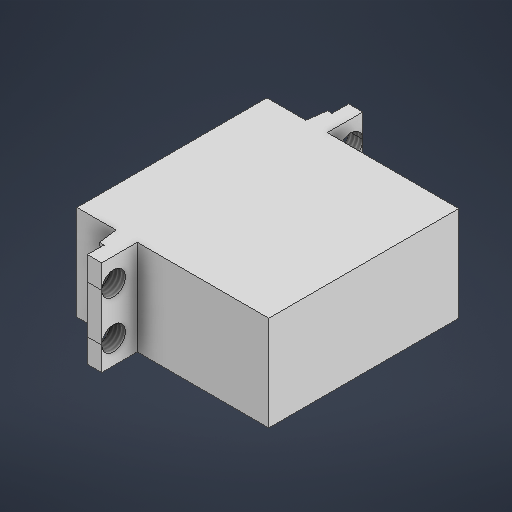
# Autodesk Inventor part: Servo
Saved by Autodesk Inventor 2026.1 (Build 301233000, 233)
## iProperties
Created: 2026-07-12
Part Number: Servo
Material: Generic
Document SubType Name: Modeling
Designer: ankit
Density: 1 g/cm^3
Appearance: Default
Author: ankit
Autodesk Inventor part; units mm, degrees
ref_plane "YZ Plane" through (0, 0, 0) normal (1, 0, 0) x (0, 1, 0)
ref_plane "XZ Plane" through (0, 0, 0) normal (0, 1, 0) x (-1, 0, 0)
ref_plane "XY Plane" through (0, 0, 0) normal (0, 0, 1) x (1, 0, 0)
sketch "Sketch1" plane through (0, 0, 0) normal (0, 1, 0) x (-1, 0, 0)
  line L0 (20.2, 20) -> (-20.2, 20)
  line L1 (-20.2, 20) -> (-20.2, -20)
  line L2 (-20.2, -20) -> (20.2, -20)
  line L3 (20.2, -20) -> (20.2, 20)
  line L4 (20.2, 20) -> (-20.2, -20) construction
  line L5 (-20.2, 20) -> (20.2, -20) construction
  line L6 (-20.2, 20) -> (7.5, 20)
  line L7 (7.5, 20) -> (7.5, 27.5)
  line L8 (7.5, 27.5) -> (10.5, 27.5)
  line L9 (10.5, 27.5) -> (10.5, 20)
  line L10 (10.5, 24) -> (11.4512, 24)
  line L11 (11.4512, 24) -> (12, 20)
  line L12 (20.2, 0) -> (-20.2, 0)
  line L13 (7.5, -20) -> (7.5, -27.5)
  line L14 (7.5, -27.5) -> (10.5, -27.5)
  line L15 (10.5, -27.5) -> (10.5, -20)
  line L16 (10.5, -24) -> (11.4512, -24)
  line L17 (11.4512, -24) -> (12, -20)
  line L18 (-20.2, -20) -> (-15.2, -20)
  line L19 (-15.2, -20) -> (-15.2, -23)
  line L20 (-15.2, -23) -> (-13.2, -23)
  line L21 (-13.2, -23) -> (-13.2, -20)
  point P0 (0, 0)
  dimension "d0" = 40.4
  dimension "d1" = 40
  dimension "d2" = 27.7
  dimension "d3" = 7.5
  dimension "d4" = 3
  dimension "d5" = 5
  dimension "d6" = 2
  constraints: 44 end point, 8 perpendicular, 7 point on line, 7 symmetric about line, 4 midpoint, 2 parallel, 1 horizontal
  measures "d0" distance of L2.end L1.end
  measures "d1" distance of L1.end L0.end
  measures "d2" distance of L0.end L6.end
  measures "d3" distance of L6.end L7.end
  measures "d4" distance of L7.end L8.end
  measures "d5" distance of L1.end L18.end
  measures "d6" distance of L19.end L20.end
extrude "Extrusion1" add sketch "Sketch1" along normal blind 20
sketch "Sketch3" plane through (-20.2, 0, -20) normal (-1, 0, 0) x (0, 0, 1)
  circle A0 centre (31, 10) radius 1.5
  line L0 (47.5, 0) -> (47.5, 20) projected
  line L1 (47.5, 10) -> (-7.5, 10)
  line L2 (-7.5, 0) -> (-7.5, 20) projected
  line L3 (20, 0) -> (20, 20)
  line L4 (0, 20) -> (40, 20) projected
  circle A1 centre (45, 5) radius 2.5
  circle A2 centre (45, 15) radius 2.5
  circle A3 centre (-5, 5) radius 2.5
  circle A4 centre (-5, 15) radius 2.5
  line L5 (45, 5) -> (45, 5)
  dimension "d24" = 0
  constraints: 6 end point, 5 centre point, 3 midpoint, 3 symmetric about line, 1 vertical, 3 other
  measures "d24" distance of L5.start L5.end
sketch "Sketch4" plane through (15.2, 0, -23) normal (0, 0, -1) x (-1, 0, 0)
  line L0 (0, 0) -> (0, 20) projected
  line L1 (4, 25) -> (0, 25)
  line L2 (0, 25) -> (0, 15)
  line L3 (0, 15) -> (4, 15)
  line L4 (4, 15) -> (4, 25)
  line L5 (2, 0) -> (2, 20) projected
  line L6 (4, 25) -> (0, 15) construction
  line L7 (0, 25) -> (4, 15) construction
  line L8 (4, -5) -> (0, -5)
  line L9 (0, -5) -> (0, 5)
  line L10 (0, 5) -> (4, 5)
  line L11 (4, 5) -> (4, -5)
  line L12 (4, -5) -> (0, 5) construction
  line L13 (0, -5) -> (4, 5) construction
  point P0 (15.2, 0)
  constraints: 24 end point, 4 midpoint, 4 parallel, 2 horizontal, 2 perpendicular, 2 point on line
extrude "Extrusion4" cut sketch "Sketch4" against normal blind 3 contours L0 L10 L11 L8 L9 | L0 L2 L1 L4 L3
extrude "Extrusion5" cut sketch "Sketch3" against normal blind 15 contours A3 | A4 | A2 | A1
extrude "Extrusion6" add sketch "Sketch3" along normal blind 5 contours L1 A0 | A0 L1
thread "Thread1" size "M5x0.8" class "6H" standard "ANSI Metric M Profile" full length
thread "Thread2" size "M5x0.8" class "6H" standard "ANSI Metric M Profile" full length
thread "Thread3" size "M5x0.8" class "6H" standard "ANSI Metric M Profile" full length
thread "Thread4" size "M5x0.8" class "6H" standard "ANSI Metric M Profile" full length
sketch "Sketch5" plane through (-20.2, 0, -20) normal (-1, 0, 0) x (0, 0, 1)
  circle A0 centre (45, 15) radius 4.5
  circle A1 centre (45, 5) radius 4.5
  circle A2 centre (-5, 5) radius 2.5 projected
  circle A3 centre (-5, 5) radius 4.5
  circle A4 centre (-5, 15) radius 2.5 projected
  circle A5 centre (-5, 15) radius 4.5
  point P0 (20, 0)
  point P1 (-7.5, 5)
  point P2 (-7.5, 15)
  dimension "d33" = 9
  dimension "d34" = 9
  dimension "d35" = 9
  dimension "d36" = 9
  constraints: 4 centre point, 2 coincident, 2 horizontal alignment
  measures "d33" diameter of A0
  measures "d34" diameter of A1
  measures "d35" diameter of A3
  measures "d36" diameter of A5
extrude "Extrusion7" cut sketch "Sketch5" against normal blind 9.6 contours A0 | A1 | A2 | A3 | A5
body "Solid1"
